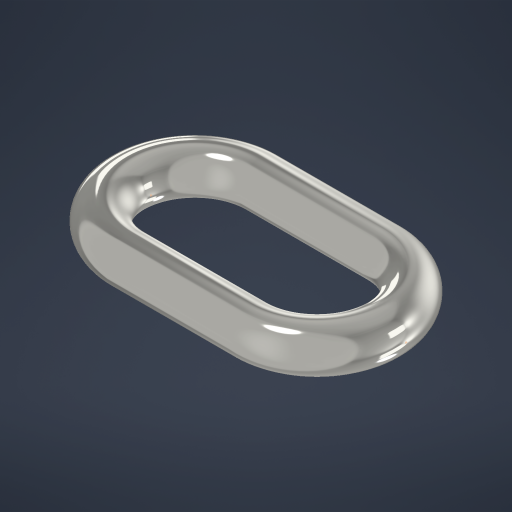
# Autodesk Inventor part: cadena
Saved by Autodesk Inventor 2024 (Build 280153000, 153)
## iProperties
Created: 2015-11-26
Part Number: cadena
Material: Acero
Document SubType Name: Modeling
Designer: H. Valenzuela B.
Density: 7.85 g/cm^3
Appearance: Plata
Author: H. Valenzuela B.
Autodesk Inventor part; units mm, degrees
ref_plane "YZ Plane" through (0, 0, 0) normal (1, 0, 0) x (0, 1, 0)
ref_plane "XZ Plane" through (0, 0, 0) normal (0, 1, 0) x (-1, 0, 0)
sketch "Boceto2" plane through (0, 0, 0) normal (1, 0, 0) x (0, 1, 0)
  circle A0 centre (6, 0) radius 2
  point P0 (0, 0)
  dimension "d4" = 4
  constraints: 1 centre point, 1 coincident
  measures "d4" diameter of A0
sketch "Boceto1" plane through (0, 0, 0) normal (0, 0, 1) x (1, 0, 0)
  line L0 (-5.5, 0) -> (5.5, 0) construction
  line L1 (-5.5, -8) -> (5.5, -8)
  line L2 (5.5, 8) -> (-5.5, 8)
  arc A0 (-5.5, 8) -> (-5.5, -8) centre (-5.5, 0) ccw
  arc A1 (5.5, -8) -> (5.5, 8) centre (5.5, 0) ccw
  line L3 (-5.5, 0) -> (5.5, 0) construction
  line L4 (-5.5, -4) -> (5.5, -4)
  line L5 (5.5, 4) -> (-5.5, 4)
  arc A2 (-5.5, 4) -> (-5.5, -4) centre (-5.5, 0) ccw
  arc A3 (5.5, -4) -> (5.5, 4) centre (5.5, 0) ccw
  line L6 (-5.5, 6) -> (5.5, 6)
  arc A4 (5.5, -6) -> (5.5, 6) centre (5.5, 0) ccw
  line L7 (5.5, -6) -> (-5.5, -6)
  arc A5 (-5.5, 6) -> (-5.5, -6) centre (-5.5, 0) ccw
  point P0 (0, 0)
  dimension "d0" = 16
  dimension "d1" = 4
  dimension "d2" = 19
  dimension "d3" = 2
  constraints: 20 end point, 12 point on circle, 8 tangent, 6 centre point, 3 parallel, 2 midpoint, 1 horizontal, 1 point on line, 3 other
  measures "d0" distance between parallel lines of L1 L2
  measures "d1" distance between parallel lines of L1 L4
  measures "d3" distance between parallel lines of L2 L6
sweep "Barrido1" add profiles "Boceto2" path "Boceto1" path curves L6 A4 L7 A5
ref_plane "Plano de trabajo1" through (-5.5, 0, 0) normal (0, 0, -1) x (-1, 0, 0)
sketch "Boceto3" plane through (-5.5, 0, 0) normal (0, 0, -1) x (-1, 0, 0)
  arc A0 (-11, 8) -> (-11, -8) centre (-11, 0) ccw projected
  point P0 (-5.5, 0)
  point P1 (4, 0)
  point P2 (-15, 0)
  point P3 (8, 0)
  point P4 (-19, 0)
  constraints: 1 point on circle
